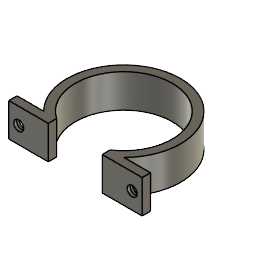
clamp (Autodesk Fusion 360 design; units mm, degrees)
part number: 2026-05-16-11-32-00-611
Autodesk Fusion 360 part; units mm, degrees
sketch "Sketch1" plane through (0, 0, 0) normal (0, 0, 1) x (1, 0, 0)
  line L0 (0, 0) -> (0, 14.5)
  circle A0 centre (0, 14.5) radius 14.5
  circle A1 centre (0, 14.5) radius 17
  line L1 (-8.8664, -0.0047) -> (8.8664, -0.0047)
  line L2 (20, 0) -> (8, 0)
  line L3 (8, 0) -> (8, 2.5)
  line L4 (8, 2.5) -> (20, 2.5)
  line L5 (20, 2.5) -> (20, 0)
  line L6 (0, 33) -> (0, -5) construction
  line L7 (-20, 0) -> (-8.1394, 0)
  line L8 (-8.1394, 0) -> (-8.1394, 2.5)
  line L9 (-8.1394, 2.5) -> (-20, 2.5)
  line L10 (-20, 2.5) -> (-20, 0)
  dimension "d2" = 14.5
  dimension "d3" = 29
  dimension "d4" = 34
  dimension "d5" = 2.5
  constraint coincident L0.start origin
  constraint vertical L0
  constraint coincident L0.end A0.centre
  constraint concentric A0 A1
  constraint coincident A1 L1.start
  constraint coincident A1 L1.end
  constraint perpendicular L0 L1
  constraint horizontal L2
  constraint vertical L3
  constraint horizontal L4
  constraint vertical L5
  constraint perpendicular L1 L6
  constraint horizontal L7
  constraint vertical L8
  constraint horizontal L9
  constraint vertical L10
  constraint coincident A0 L8.end
  measures "d2" distance of L0.start L0.end
  measures "d3" diameter of A0
  measures "d4" diameter of A1
  measures "d5" distance of L7.start L9.end
extrude "Extrude1" add sketch "Sketch1" along normal blind 10 contours A0 A1 L4 L9 | A1 L7 L8 L9 | A0 A1 L2 L3 L4 | A1 L7 L9 L10 | A1 L2 L4 L5
sketch "Sketch2" plane through (0, 2.5, 0) normal (0, 1, 0) x (-1, 0, 0)
  line L0 (-20, 0) -> (-12.0416, 0)
  line L1 (-12.0416, 0) -> (-12.0416, 10)
  line L2 (-12.0416, 10) -> (-20, 10)
  line L3 (-20, 10) -> (-20, 0)
  point P0 (-17, 5)
  point P1 (17, 5)
hole "Hole1" at (17, 2.5, 5) at (-17, 2.5, 5) direction (0, -1, 0) diameter 3 depth 2.5 tip angle 180 counterbore diameter 5.5 counterbore depth 1.6
